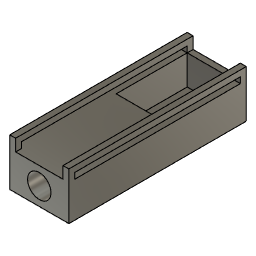
Chalk Holder Final (Autodesk Fusion 360 design; units mm, degrees)
Autodesk Fusion 360 part; units mm, degrees
sketch "Sketch2" plane through (0, 0, 0) normal (0, -1, 0) x (1, 0, 0)
  line L0 (-25, 15) -> (-25, 0)
  line L1 (-25, 0) -> (0, 0)
  line L2 (0, 0) -> (0, 15)
  line L3 (0, 15) -> (-25, 15)
  circle A0 centre (-12.5, 7.5) radius 4.965
  dimension "d7" = 9.93
  measures "d7" diameter of A0
box "BoxPrimitive2" add length 15 width 25 height 75 placed x (0, 0, 1) y (1, 0, 0) z (0, 1, 0) at (-25, 0, 0) makes body 1
extrude "Extrude1" cut sketch "Sketch2" against normal blind 40 contours A0 bodies 1
box "BoxPrimitive3" add length 30 width 20 height 12.5 placed x (0, -1, 0) y (1, 0, 0) z (0, 0, 1) at (-25, 75, 0) separate body makes body 2
move_body "Move1" bodies 2 to x (1, 0, 0) y (0, 1, 0) z (0, 0, 1) at (2.5, -2.5, 2.5)
combine "Combine1" operation cut target body 1 tool bodies 2
box "BoxPrimitive4" add length 2.5 width 2.5 height 20 placed x (0, 1, 0) y (-1, 0, 0) z (0, 0, 1) at (0, 0, 0) separate body makes body 3
copy_body "CopyPasteBodies1" bodies 3 makes body 4
move_body "Move2" bodies 4 to x (1, 0, 0) y (0, 1, 0) z (0, 0, 1) at (-22.5, 0, 0)
copy_body "CopyPasteBodies2" bodies 3 4 makes body 5 makes body 6
move_body "Move3" bodies 5 6 to x (1, 0, 0) y (0, 1, 0) z (0, 0, 1) at (0, 72.5, 0)
box "BoxPrimitive5" add length 75 width 2.5 height 2.5 placed x (0, 1, 0) y (-1, 0, 0) z (0, 0, 1) at (0, 0, 0) separate body makes body 7
move_body "Move4" bodies 7 to x (1, 0, 0) y (0, 1, 0) z (0, 0, 1) at (0, 0, 17.5)
copy_body "CopyPasteBodies3" bodies 7 makes body 8
move_body "Move5" bodies 8 to x (1, 0, 0) y (0, 1, 0) z (0, 0, 1) at (-22.5, 0, 0)
combine "Combine2" operation add target body 1 tool bodies 6 8 7 3 5 4
